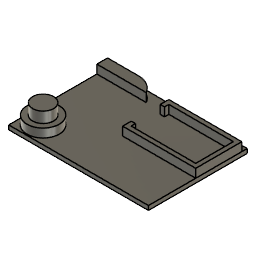
Kurbelschleifen_Funktionstester (Autodesk Fusion 360 design; units mm, degrees)
Autodesk Fusion 360 part; units mm, degrees
box "Grundkörper Quader1" add length 46 width 65 height 2 placed x (0, -1, 0) y (1, 0, 0) z (0, 0, 1) at (2, -2, 0) makes body 1
cylinder "Grundkörper Zylinder1" add diameter 9.8 height 9 placed x (1, 0, 0) y (0, 1, 0) z (0, 0, 1) at (10, -40, 2) bodies 1
box "Grundkörper Quader2" add length 17.5 width 30 height 4 placed x (0, -1, 0) y (1, 0, 0) z (0, 0, 1) at (35, -6.5, 2) separate body makes body 2
shell "Schale1" thickness 2 outward yes removed faces 2 at (55, -12.3333, 6) at (55, -12.3333, 2) on bodies 2
sketch "Skizze11" plane through (0, 0, 6) normal (0, 0, 1) x (-1, 0, 0)
  line L0 (-35, 24) -> (-35, 6.5)
  line L1 (-35, 6.5) -> (-65, 6.5)
  line L2 (-65, 6.5) -> (-65, 24)
  line L3 (-65, 24) -> (-35, 24)
  line L4 (-33, 26) -> (-67, 26)
  line L5 (-67, 26) -> (-67, 4.5)
  line L6 (-67, 4.5) -> (-33, 4.5)
  line L7 (-33, 4.5) -> (-33, 26)
  line L8 (-33, 8.5) -> (-35, 8.5)
  line L9 (-35, 8.5) -> (-35, 22)
  line L10 (-35, 22) -> (-33, 22)
  line L11 (-33, 22) -> (-33, 8.5)
  dimension "d17" = 4
  dimension "d18" = 4
  constraint horizontal L8
  constraint vertical L9
  constraint horizontal L10
  constraint vertical L11
  constraint coincident L0 L9.end
  constraint coincident L7 L8.start
  measures "d17" distance of L6 L8
  measures "d18" distance of L4 L10
extrude "Extrusion1" cut sketch "Skizze11" against normal blind 4 contours L0 L7 L8 L9 L10 L11 bodies 2
sketch "Skizze13" plane through (0, 0, 2) normal (0, 0, 1) x (-1, 0, 0)
  circle A0 centre (-10, 40) radius 4.9
  line L0 (-2, 48) -> (-67, 48)
  line L1 (-67, 48) -> (-67, 2)
  line L2 (-67, 2) -> (-2, 2)
  line L3 (-2, 2) -> (-2, 48)
  circle A1 centre (-10, 40) radius 7.5
  line L4 (-2, 2) -> (-25, 2)
  line L5 (-25, 2) -> (-25, 7)
  line L6 (-25, 7) -> (-2, 7)
  line L7 (-2, 7) -> (-2, 2)
  dimension "d25" = 15
  constraint concentric A0 A1
  constraint horizontal L4
  constraint vertical L5
  constraint horizontal L6
  constraint vertical L7
  measures "d25" diameter of A1
extrude "Extrusion2" add sketch "Skizze13" along normal blind 4 contours A1 bodies 1
extrude "Extrusion3" add sketch "Skizze13" along normal blind 4 contours L2 L3 L4 L5 L6 L7 bodies 1
fillet "Abrundung1" radius 10 1 edges at (25, -2, 4) on bodies 1
